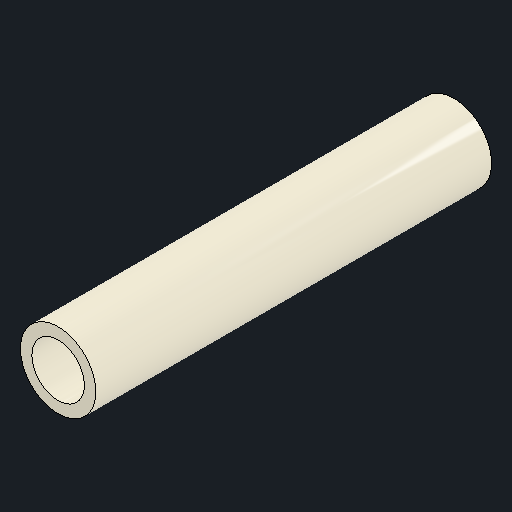
# Autodesk Inventor part: ignition-alumina-tube-lower
Saved by Autodesk Inventor 2027.1 (Build 311270010, 270A)
## iProperties
Created: 2026-10-02
Part Number: ignition-alumina-tube-lower
Material: Alumina
Description: Alumina ignition clamp tube; provisional OD 6 mm, bore 3.2 mm, length 24.187373 mm. Physical material properties require verification.
Document SubType Name: Modeling
Designer: queezz
Density: 1 g/cm^3
Appearance: Alumina ivory
Author: queezz
Autodesk Inventor part; units mm, degrees
ref_plane "YZ Plane" through (0, 0, 0) normal (1, 0, 0) x (0, 1, 0)
ref_plane "XZ Plane" through (0, 0, 0) normal (0, 1, 0) x (-1, 0, 0)
ref_plane "XY Plane" through (0, 0, 0) normal (0, 0, 1) x (1, 0, 0)
sketch "Tube OD 6 mm - bore 3.2 mm" plane through (0, 0, 0) normal (0, 0, 1) x (1, 0, 0)
  circle A0 centre (0, 0) radius 2.3
  circle A1 centre (0, 0) radius 1.6
  dimension "d2" = 4.6
  dimension "d3" = 3.2
  constraints: 2 centre point, 2 coincident
  measures "d2" diameter of A0
  measures "d3" diameter of A1
extrude "Tube length" add sketch "Tube OD 6 mm - bore 3.2 mm" along normal blind 24.1874
body "Solid1"
